Autodesk Fusion 360 part; units mm, degrees
(part 3 of 15)
  spline S34 degree 5 poles (-13.0691, -22.8361) (-13.0745, -22.8455) (-13.085, -22.8643) (-13.1, -22.893) (-13.1188, -22.9319) (-13.1404, -22.9814) (-13.1608, -23.0315) (-13.1803, -23.0821) (-13.1994, -23.133) (-13.2182, -23.1839) (-13.2367, -23.2351) (-13.2548, -23.2864) (-13.2724, -23.338) (-13.2894, -23.3899) (-13.3057, -23.4421) (-13.3214, -23.4946) (-13.3366, -23.5473) (-13.3514, -23.6002) (-13.3658, -23.6533) (-13.3798, -23.7066) (-13.3935, -23.76) (-13.4069, -23.8135) (-13.4198, -23.8673) (-13.4324, -23.9212) (-13.4445, -23.9753) (-13.4563, -24.0295) (-13.4677, -24.0839) (-13.4788, -24.1385) (-13.4895, -24.1932) (-13.4999, -24.248) (-13.51, -24.3029) (-13.5197, -24.358) (-13.5291, -24.4132) (-13.5382, -24.4686) (-13.547, -24.524) (-13.5555, -24.5796) (-13.5636, -24.6353) (-13.5714, -24.6912) (-13.579, -24.7471) (-13.5862, -24.8032) (-13.5932, -24.8593) (-13.5998, -24.9156) (-13.6062, -24.972) (-13.6123, -25.0284) (-13.618, -25.085) (-13.6235, -25.1417) (-13.6288, -25.1985) (-13.6337, -25.2553) (-13.6383, -25.3123) (-13.6427, -25.3694) (-13.6468, -25.4265) (-13.6507, -25.4838) (-13.6542, -25.5411) (-13.6575, -25.5985) (-13.6606, -25.656) (-13.6633, -25.7136) (-13.6659, -25.7712) (-13.6681, -25.829) (-13.6701, -25.8868) (-13.6718, -25.9447) (-13.6733, -26.0027) (-13.6745, -26.0607) (-13.6754, -26.1188) (-13.6761, -26.177) (-13.6766, -26.2353) (-13.6768, -26.2936) (-13.6767, -26.3521) (-13.6765, -26.4105) (-13.6759, -26.4691) (-13.6751, -26.5277) (-13.6741, -26.5863) (-13.6731, -26.6333) (-13.6722, -26.6686) (-13.6715, -26.6921) (-13.6712, -26.7039) knots 0 0 0 0 0 0 0.01428571 0.02857143 0.04285714 0.05714286 0.07142857 0.08571429 0.1 0.11428571 0.12857143 0.14285714 0.15714286 0.17142857 0.18571429 0.2 0.21428571 0.22857143 0.24285714 0.25714286 0.27142857 0.28571429 0.3 0.31428571 0.32857143 0.34285714 0.35714286 0.37142857 0.38571429 0.4 0.41428571 0.42857143 0.44285714 0.45714286 0.47142857 0.48571429 0.5 0.51428571 0.52857143 0.54285714 0.55714286 0.57142857 0.58571429 0.6 0.61428571 0.62857143 0.64285714 0.65714286 0.67142857 0.68571429 0.7 0.71428571 0.72857143 0.74285714 0.75714286 0.77142857 0.78571429 0.8 0.81428571 0.82857143 0.84285714 0.85714286 0.87142857 0.88571429 0.9 0.91428571 0.92857143 0.94285714 0.95714286 0.97142857 0.98571429 1 1 1 1 1 1
  arc A36 (-13.6712, -26.7039) -> (-12.3541, -27.3382) centre (0, 0) ccw
  spline S35 degree 5 poles (-9.7055, -24.4559) (-9.7095, -24.466) (-9.7177, -24.4859) (-9.7307, -24.5156) (-9.7494, -24.5545) (-9.7746, -24.6023) (-9.8012, -24.6494) (-9.8286, -24.6963) (-9.8564, -24.7429) (-9.8845, -24.7894) (-9.9129, -24.8357) (-9.9418, -24.8819) (-9.9712, -24.9278) (-10.0012, -24.9734) (-10.0318, -25.0187) (-10.0631, -25.0637) (-10.0948, -25.1085) (-10.127, -25.153) (-10.1595, -25.1974) (-10.1924, -25.2416) (-10.2256, -25.2856) (-10.2591, -25.3294) (-10.2931, -25.3731) (-10.3274, -25.4165) (-10.3621, -25.4597) (-10.3972, -25.5027) (-10.4326, -25.5456) (-10.4683, -25.5882) (-10.5044, -25.6307) (-10.5408, -25.673) (-10.5775, -25.7151) (-10.6145, -25.7571) (-10.6518, -25.7989) (-10.6894, -25.8405) (-10.7273, -25.882) (-10.7654, -25.9232) (-10.8039, -25.9643) (-10.8427, -26.0053) (-10.8817, -26.0461) (-10.921, -26.0867) (-10.9606, -26.1271) (-11.0004, -26.1674) (-11.0406, -26.2075) (-11.0809, -26.2475) (-11.1216, -26.2873) (-11.1624, -26.3269) (-11.2036, -26.3664) (-11.245, -26.4057) (-11.2866, -26.4449) (-11.3285, -26.4839) (-11.3706, -26.5227) (-11.4129, -26.5614) (-11.4555, -26.5999) (-11.4984, -26.6383) (-11.5414, -26.6765) (-11.5847, -26.7146) (-11.6282, -26.7525) (-11.672, -26.7902) (-11.716, -26.8279) (-11.7601, -26.8653) (-11.8046, -26.9026) (-11.8492, -26.9397) (-11.894, -26.9767) (-11.9391, -27.0136) (-11.9844, -27.0502) (-12.0299, -27.0868) (-12.0755, -27.1231) (-12.1215, -27.1594) (-12.1676, -27.1954) (-12.2139, -27.2314) (-12.2604, -27.2671) (-12.2978, -27.2956) (-12.3259, -27.3169) (-12.3447, -27.3311) (-12.3541, -27.3382) knots 0 0 0 0 0 0 0.01428571 0.02857143 0.04285714 0.05714286 0.07142857 0.08571429 0.1 0.11428571 0.12857143 0.14285714 0.15714286 0.17142857 0.18571429 0.2 0.21428571 0.22857143 0.24285714 0.25714286 0.27142857 0.28571429 0.3 0.31428571 0.32857143 0.34285714 0.35714286 0.37142857 0.38571429 0.4 0.41428571 0.42857143 0.44285714 0.45714286 0.47142857 0.48571429 0.5 0.51428571 0.52857143 0.54285714 0.55714286 0.57142857 0.58571429 0.6 0.61428571 0.62857143 0.64285714 0.65714286 0.67142857 0.68571429 0.7 0.71428571 0.72857143 0.74285714 0.75714286 0.77142857 0.78571429 0.8 0.81428571 0.82857143 0.84285714 0.85714286 0.87142857 0.88571429 0.9 0.91428571 0.92857143 0.94285714 0.95714286 0.97142857 0.98571429 1 1 1 1 1 1
  line L35 (-9.7055, -24.4559) -> (-9.4748, -23.8746)
  arc A37 (-9.4748, -23.8746) -> (-7.4779, -24.5734) centre (0, 0) ccw
  line L36 (-7.4779, -24.5734) -> (-7.6599, -25.1717)
  spline S36 degree 5 poles (-7.6599, -25.1717) (-7.6631, -25.182) (-7.6691, -25.2028) (-7.6774, -25.2341) (-7.6871, -25.2761) (-7.6971, -25.3292) (-7.7058, -25.3826) (-7.7136, -25.4363) (-7.7209, -25.4901) (-7.7279, -25.544) (-7.7346, -25.598) (-7.7408, -25.6521) (-7.7465, -25.7063) (-7.7514, -25.7606) (-7.7557, -25.8152) (-7.7594, -25.8698) (-7.7625, -25.9246) (-7.7651, -25.9795) (-7.7673, -26.0345) (-7.7692, -26.0895) (-7.7706, -26.1446) (-7.7717, -26.1998) (-7.7724, -26.2551) (-7.7726, -26.3104) (-7.7725, -26.3659) (-7.7719, -26.4214) (-7.7709, -26.4769) (-7.7695, -26.5326) (-7.7678, -26.5883) (-7.7657, -26.644) (-7.7633, -26.6999) (-7.7606, -26.7557) (-7.7575, -26.8117) (-7.754, -26.8676) (-7.7502, -26.9237) (-7.7461, -26.9797) (-7.7417, -27.0359) (-7.7369, -27.092) (-7.7318, -27.1483) (-7.7264, -27.2045) (-7.7206, -27.2608) (-7.7146, -27.3172) (-7.7083, -27.3735) (-7.7016, -27.4299) (-7.6947, -27.4864) (-7.6874, -27.5429) (-7.6799, -27.5994) (-7.672, -27.6559) (-7.6639, -27.7125) (-7.6555, -27.7691) (-7.6468, -27.8257) (-7.6378, -27.8824) (-7.6285, -27.9391) (-7.6189, -27.9958) (-7.6091, -28.0525) (-7.599, -28.1093) (-7.5886, -28.166) (-7.5779, -28.2228) (-7.567, -28.2796) (-7.5558, -28.3365) (-7.5443, -28.3933) (-7.5326, -28.4502) (-7.5206, -28.5071) (-7.5083, -28.564) (-7.4958, -28.6209) (-7.483, -28.6778) (-7.47, -28.7347) (-7.4567, -28.7917) (-7.4431, -28.8486) (-7.4293, -28.9056) (-7.4152, -28.9625) (-7.4038, -29.0081) (-7.3951, -29.0423) (-7.3892, -29.0651) (-7.3863, -29.0765) knots 0 0 0 0 0 0 0.01428571 0.02857143 0.04285714 0.05714286 0.07142857 0.08571429 0.1 0.11428571 0.12857143 0.14285714 0.15714286 0.17142857 0.18571429 0.2 0.21428571 0.22857143 0.24285714 0.25714286 0.27142857 0.28571429 0.3 0.31428571 0.32857143 0.34285714 0.35714286 0.37142857 0.38571429 0.4 0.41428571 0.42857143 0.44285714 0.45714286 0.47142857 0.48571429 0.5 0.51428571 0.52857143 0.54285714 0.55714286 0.57142857 0.58571429 0.6 0.61428571 0.62857143 0.64285714 0.65714286 0.67142857 0.68571429 0.7 0.71428571 0.72857143 0.74285714 0.75714286 0.77142857 0.78571429 0.8 0.81428571 0.82857143 0.84285714 0.85714286 0.87142857 0.88571429 0.9 0.91428571 0.92857143 0.94285714 0.95714286 0.97142857 0.98571429 1 1 1 1 1 1
  arc A38 (-7.3863, -29.0765) -> (-5.961, -29.4018) centre (0, 0) ccw
  spline S37 degree 5 poles (-4.0202, -26.0024) (-4.0219, -26.0131) (-4.0254, -26.0344) (-4.0315, -26.0662) (-4.0411, -26.1083) (-4.055, -26.1605) (-4.0704, -26.2124) (-4.0867, -26.2641) (-4.1034, -26.3158) (-4.1205, -26.3674) (-4.1379, -26.4189) (-4.1558, -26.4703) (-4.1742, -26.5216) (-4.1933, -26.5728) (-4.2131, -26.6237) (-4.2336, -26.6746) (-4.2545, -26.7253) (-4.276, -26.7759) (-4.2978, -26.8263) (-4.32, -26.8767) (-4.3426, -26.927) (-4.3656, -26.9772) (-4.389, -27.0273) (-4.4128, -27.0773) (-4.437, -27.1272) (-4.4616, -27.1769) (-4.4866, -27.2266) (-4.512, -27.2761) (-4.5377, -27.3255) (-4.5637, -27.3749) (-4.5901, -27.4241) (-4.6168, -27.4733) (-4.6439, -27.5223) (-4.6713, -27.5712) (-4.699, -27.6201) (-4.7271, -27.6688) (-4.7554, -27.7175) (-4.7841, -27.766) (-4.8131, -27.8144) (-4.8424, -27.8628) (-4.872, -27.911) (-4.9018, -27.9591) (-4.932, -28.0072) (-4.9625, -28.0551) (-4.9932, -28.103) (-5.0243, -28.1507) (-5.0556, -28.1983) (-5.0872, -28.2459) (-5.1191, -28.2933) (-5.1512, -28.3407) (-5.1836, -28.3879) (-5.2163, -28.4351) (-5.2493, -28.4821) (-5.2825, -28.529) (-5.316, -28.5759) (-5.3497, -28.6226) (-5.3837, -28.6693) (-5.418, -28.7158) (-5.4525, -28.7623) (-5.4872, -28.8086) (-5.5222, -28.8548) (-5.5574, -28.901) (-5.5929, -28.947) (-5.6287, -28.993) (-5.6647, -29.0388) (-5.7009, -29.0845) (-5.7373, -29.1302) (-5.774, -29.1757) (-5.8109, -29.2211) (-5.8481, -29.2665) (-5.8855, -29.3117) (-5.9156, -29.3478) (-5.9383, -29.3748) (-5.9534, -29.3928) (-5.961, -29.4018) knots 0 0 0 0 0 0 0.01428571 0.02857143 0.04285714 0.05714286 0.07142857 0.08571429 0.1 0.11428571 0.12857143 0.14285714 0.15714286 0.17142857 0.18571429 0.2 0.21428571 0.22857143 0.24285714 0.25714286 0.27142857 0.28571429 0.3 0.31428571 0.32857143 0.34285714 0.35714286 0.37142857 0.38571429 0.4 0.41428571 0.42857143 0.44285714 0.45714286 0.47142857 0.48571429 0.5 0.51428571 0.52857143 0.54285714 0.55714286 0.57142857 0.58571429 0.6 0.61428571 0.62857143 0.64285714 0.65714286 0.67142857 0.68571429 0.7 0.71428571 0.72857143 0.74285714 0.75714286 0.77142857 0.78571429 0.8 0.81428571 0.82857143 0.84285714 0.85714286 0.87142857 0.88571429 0.9 0.91428571 0.92857143 0.94285714 0.95714286 0.97142857 0.98571429 1 1 1 1 1 1
  line L37 (-4.0202, -26.0024) -> (-3.9247, -25.3844)
  arc A39 (-3.9247, -25.3844) -> (-1.8223, -25.6213) centre (0, 0) ccw
  line L38 (-1.8223, -25.6213) -> (-1.8667, -26.2451)
  spline S38 degree 5 poles (-1.8667, -26.2451) (-1.8674, -26.2559) (-1.8687, -26.2774) (-1.8698, -26.3098) (-1.8699, -26.3529) (-1.8679, -26.4069) (-1.8644, -26.461) (-1.8601, -26.515) (-1.8552, -26.5691) (-1.8501, -26.6232) (-1.8446, -26.6773) (-1.8386, -26.7314) (-1.8321, -26.7855) (-1.8248, -26.8396) (-1.8169, -26.8937) (-1.8082, -26.9478) (-1.7991, -27.0019) (-1.7894, -27.056) (-1.7794, -27.1101) (-1.7689, -27.1642) (-1.7581, -27.2182) (-1.7469, -27.2723) (-1.7352, -27.3263) (-1.7231, -27.3803) (-1.7106, -27.4343) (-1.6977, -27.4883) (-1.6844, -27.5423) (-1.6707, -27.5962) (-1.6566, -27.6502) (-1.6422, -27.7041) (-1.6274, -27.7579) (-1.6123, -27.8118) (-1.5968, -27.8656) (-1.581, -27.9194) (-1.5648, -27.9732) (-1.5483, -28.027) (-1.5315, -28.0807) (-1.5143, -28.1344) (-1.4969, -28.1881) (-1.4791, -28.2417) (-1.461, -28.2953) (-1.4425, -28.3489) (-1.4238, -28.4025) (-1.4048, -28.456) (-1.3854, -28.5095) (-1.3658, -28.5629) (-1.3459, -28.6163) (-1.3256, -28.6697) (-1.3051, -28.7231) (-1.2843, -28.7764) (-1.2632, -28.8296) (-1.2418, -28.8829) (-1.2202, -28.9361) (-1.1983, -28.9892) (-1.176, -29.0423) (-1.1536, -29.0954) (-1.1308, -29.1485) (-1.1078, -29.2015) (-1.0845, -29.2544) (-1.0609, -29.3073) (-1.0371, -29.3602) (-1.013, -29.413) (-0.9886, -29.4658) (-0.964, -29.5186) (-0.9391, -29.5712) (-0.914, -29.6239) (-0.8886, -29.6765) (-0.863, -29.729) (-0.8371, -29.7816) (-0.8109, -29.834) (-0.7845, -29.8864) (-0.7632, -29.9283) (-0.7471, -29.9597) (-0.7364, -29.9806) (-0.731, -29.9911) knots 0 0 0 0 0 0 0.01428571 0.02857143 0.04285714 0.05714286 0.07142857 0.08571429 0.1 0.11428571 0.12857143 0.14285714 0.15714286 0.17142857 0.18571429 0.2 0.21428571 0.22857143 0.24285714 0.25714286 0.27142857 0.28571429 0.3 0.31428571 0.32857143 0.34285714 0.35714286 0.37142857 0.38571429 0.4 0.41428571 0.42857143 0.44285714 0.45714286 0.47142857 0.48571429 0.5 0.51428571 0.52857143 0.54285714 0.55714286 0.57142857 0.58571429 0.6 0.61428571 0.62857143 0.64285714 0.65714286 0.67142857 0.68571429 0.7 0.71428571 0.72857143 0.74285714 0.75714286 0.77142857 0.78571429 0.8 0.81428571 0.82857143 0.84285714 0.85714286 0.87142857 0.88571429 0.9 0.91428571 0.92857143 0.94285714 0.95714286 0.97142857 0.98571429 1 1 1 1 1 1
  arc A40 (-0.731, -29.9911) -> (0.731, -29.9911) centre (0, 0) ccw
  spline S39 degree 5 poles (1.8667, -26.2451) (1.8674, -26.2559) (1.8687, -26.2774) (1.8698, -26.3098) (1.8699, -26.3529) (1.8679, -26.4069) (1.8644, -26.461) (1.8601, -26.515) (1.8552, -26.5691) (1.8501, -26.6232) (1.8446, -26.6773) (1.8386, -26.7314) (1.8321, -26.7855) (1.8248, -26.8396) (1.8169, -26.8937) (1.8082, -26.9478) (1.7991, -27.0019) (1.7894, -27.056) (1.7794, -27.1101) (1.7689, -27.1642) (1.7581, -27.2182) (1.7469, -27.2723) (1.7352, -27.3263) (1.7231, -27.3803) (1.7106, -27.4343) (1.6977, -27.4883) (1.6844, -27.5423) (1.6707, -27.5962) (1.6566, -27.6502) (1.6422, -27.7041) (1.6274, -27.7579) (1.6123, -27.8118) (1.5968, -27.8656) (1.581, -27.9194) (1.5648, -27.9732) (1.5483, -28.027) (1.5315, -28.0807) (1.5143, -28.1344) (1.4969, -28.1881) (1.4791, -28.2417) (1.461, -28.2953) (1.4425, -28.3489) (1.4238, -28.4025) (1.4048, -28.456) (1.3854, -28.5095) (1.3658, -28.5629) (1.3459, -28.6163) (1.3256, -28.6697) (1.3051, -28.7231) (1.2843, -28.7764) (1.2632, -28.8296) (1.2418, -28.8829) (1.2202, -28.9361) (1.1983, -28.9892) (1.176, -29.0423) (1.1536, -29.0954) (1.1308, -29.1485) (1.1078, -29.2015) (1.0845, -29.2544) (1.0609, -29.3073) (1.0371, -29.3602) (1.013, -29.413) (0.9886, -29.4658) (0.964, -29.5186) (0.9391, -29.5712) (0.914, -29.6239) (0.8886, -29.6765) (0.863, -29.729) (0.8371, -29.7816) (0.8109, -29.834) (0.7845, -29.8864) (0.7632, -29.9283) (0.7471, -29.9597) (0.7364, -29.9806) (0.731, -29.9911) knots 0 0 0 0 0 0 0.01428571 0.02857143 0.04285714 0.05714286 0.07142857 0.08571429 0.1 0.11428571 0.12857143 0.14285714 0.15714286 0.17142857 0.18571429 0.2 0.21428571 0.22857143 0.24285714 0.25714286 0.27142857 0.28571429 0.3 0.31428571 0.32857143 0.34285714 0.35714286 0.37142857 0.38571429 0.4 0.41428571 0.42857143 0.44285714 0.45714286 0.47142857 0.48571429 0.5 0.51428571 0.52857143 0.54285714 0.55714286 0.57142857 0.58571429 0.6 0.61428571 0.62857143 0.64285714 0.65714286 0.67142857 0.68571429 0.7 0.71428571 0.72857143 0.74285714 0.75714286 0.77142857 0.78571429 0.8 0.81428571 0.82857143 0.84285714 0.85714286 0.87142857 0.88571429 0.9 0.91428571 0.92857143 0.94285714 0.95714286 0.97142857 0.98571429 1 1 1 1 1 1
  line L39 (1.8667, -26.2451) -> (1.8223, -25.6213)
  arc A41 (1.8223, -25.6213) -> (3.9247, -25.3844) centre (0, 0) ccw
  line L40 (3.9247, -25.3844) -> (4.0202, -26.0024)
  spline S40 degree 5 poles (4.0202, -26.0024) (4.0219, -26.0131) (4.0254, -26.0344) (4.0315, -26.0662) (4.0411, -26.1083) (4.055, -26.1605) (4.0704, -26.2124) (4.0867, -26.2641) (4.1034, -26.3158) (4.1205, -26.3674) (4.1379, -26.4189) (4.1558, -26.4703) (4.1742, -26.5216) (4.1933, -26.5728) (4.2131, -26.6237) (4.2336, -26.6746) (4.2545, -26.7253) (4.276, -26.7759) (4.2978, -26.8263) (4.32, -26.8767) (4.3426, -26.927) (4.3656, -26.9772) (4.389, -27.0273) (4.4128, -27.0773) (4.437, -27.1272) (4.4616, -27.1769) (4.4866, -27.2266) (4.512, -27.2761) (4.5377, -27.3255) (4.5637, -27.3749) (4.5901, -27.4241) (4.6168, -27.4733) (4.6439, -27.5223) (4.6713, -27.5712) (4.699, -27.6201) (4.7271, -27.6688) (4.7554, -27.7175) (4.7841, -27.766) (4.8131, -27.8144) (4.8424, -27.8628) (4.872, -27.911) (4.9018, -27.9591) (4.932, -28.0072) (4.9625, -28.0551) (4.9932, -28.103) (5.0243, -28.1507) (5.0556, -28.1983) (5.0872, -28.2459) (5.1191, -28.2933) (5.1512, -28.3407) (5.1836, -28.3879) (5.2163, -28.4351) (5.2493, -28.4821) (5.2825, -28.529) (5.316, -28.5759) (5.3497, -28.6226) (5.3837, -28.6693) (5.418, -28.7158) (5.4525, -28.7623) (5.4872, -28.8086) (5.5222, -28.8548) (5.5574, -28.901) (5.5929, -28.947) (5.6287, -28.993) (5.6647, -29.0388) (5.7009, -29.0845) (5.7373, -29.1302) (5.774, -29.1757) (5.8109, -29.2211) (5.8481, -29.2665) (5.8855, -29.3117) (5.9156, -29.3478) (5.9383, -29.3748) (5.9534, -29.3928) (5.961, -29.4018) knots 0 0 0 0 0 0 0.01428571 0.02857143 0.04285714 0.05714286 0.07142857 0.08571429 0.1 0.11428571 0.12857143 0.14285714 0.15714286 0.17142857 0.18571429 0.2 0.21428571 0.22857143 0.24285714 0.25714286 0.27142857 0.28571429 0.3 0.31428571 0.32857143 0.34285714 0.35714286 0.37142857 0.38571429 0.4 0.41428571 0.42857143 0.44285714 0.45714286 0.47142857 0.48571429 0.5 0.51428571 0.52857143 0.54285714 0.55714286 0.57142857 0.58571429 0.6 0.61428571 0.62857143 0.64285714 0.65714286 0.67142857 0.68571429 0.7 0.71428571 0.72857143 0.74285714 0.75714286 0.77142857 0.78571429 0.8 0.81428571 0.82857143 0.84285714 0.85714286 0.87142857 0.88571429 0.9 0.91428571 0.92857143 0.94285714 0.95714286 0.97142857 0.98571429 1 1 1 1 1 1
  arc A42 (5.961, -29.4018) -> (7.3863, -29.0765) centre (0, 0) ccw
  spline S41 degree 5 poles (7.6599, -25.1717) (7.6631, -25.182) (7.6691, -25.2028) (7.6774, -25.2341) (7.6871, -25.2761) (7.6971, -25.3292) (7.7058, -25.3826) (7.7136, -25.4363) (7.7209, -25.4901) (7.7279, -25.544) (7.7346, -25.598) (7.7408, -25.6521) (7.7465, -25.7063) (7.7514, -25.7606) (7.7557, -25.8152) (7.7594, -25.8698) (7.7625, -25.9246) (7.7651, -25.9795) (7.7673, -26.0345) (7.7692, -26.0895) (7.7706, -26.1446) (7.7717, -26.1998) (7.7724, -26.2551) (7.7726, -26.3104) (7.7725, -26.3659) (7.7719, -26.4214) (7.7709, -26.4769) (7.7695, -26.5326) (7.7678, -26.5883) (7.7657, -26.644) (7.7633, -26.6999) (7.7606, -26.7557) (7.7575, -26.8117) (7.754, -26.8676) (7.7502, -26.9237) (7.7461, -26.9797) (7.7417, -27.0359) (7.7369, -27.092) (7.7318, -27.1483) (7.7264, -27.2045) (7.7206, -27.2608) (7.7146, -27.3172) (7.7083, -27.3735) (7.7016, -27.4299) (7.6947, -27.4864) (7.6874, -27.5429) (7.6799, -27.5994) (7.672, -27.6559) (7.6639, -27.7125) (7.6555, -27.7691) (7.6468, -27.8257) (7.6378, -27.8824) (7.6285, -27.9391) (7.6189, -27.9958) (7.6091, -28.0525) (7.599, -28.1093) (7.5886, -28.166) (7.5779, -28.2228) (7.567, -28.2796) (7.5558, -28.3365) (7.5443, -28.3933) (7.5326, -28.4502) (7.5206, -28.5071) (7.5083, -28.564) (7.4958, -28.6209) (7.483, -28.6778) (7.47, -28.7347) (7.4567, -28.7917) (7.4431, -28.8486) (7.4293, -28.9056) (7.4152, -28.9625) (7.4038, -29.0081) (7.3951, -29.0423) (7.3892, -29.0651) (7.3863, -29.0765) knots 0 0 0 0 0 0 0.01428571 0.02857143 0.04285714 0.05714286 0.07142857 0.08571429 0.1 0.11428571 0.12857143 0.14285714 0.15714286 0.17142857 0.18571429 0.2 0.21428571 0.22857143 0.24285714 0.25714286 0.27142857 0.28571429 0.3 0.31428571 0.32857143 0.34285714 0.35714286 0.37142857 0.38571429 0.4 0.41428571 0.42857143 0.44285714 0.45714286 0.47142857 0.48571429 0.5 0.51428571 0.52857143 0.54285714 0.55714286 0.57142857 0.58571429 0.6 0.61428571 0.62857143 0.64285714 0.65714286 0.67142857 0.68571429 0.7 0.71428571 0.72857143 0.74285714 0.75714286 0.77142857 0.78571429 0.8 0.81428571 0.82857143 0.84285714 0.85714286 0.87142857 0.88571429 0.9 0.91428571 0.92857143 0.94285714 0.95714286 0.97142857 0.98571429 1 1 1 1 1 1
  line L41 (7.6599, -25.1717) -> (7.4779, -24.5734)
  arc A43 (7.4779, -24.5734) -> (9.4748, -23.8746) centre (0, 0) ccw
  line L42 (9.4748, -23.8746) -> (9.7055, -24.4559)
  spline S42 degree 5 poles (9.7055, -24.4559) (9.7095, -24.466) (9.7177, -24.4859) (9.7307, -24.5156) (9.7494, -24.5545) (9.7746, -24.6023) (9.8012, -24.6494) (9.8286, -24.6963) (9.8564, -24.7429) (9.8845, -24.7894) (9.9129, -24.8357) (9.9418, -24.8819) (9.9712, -24.9278) (10.0012, -24.9734) (10.0318, -25.0187) (10.0631, -25.0637) (10.0948, -25.1085) (10.127, -25.153) (10.1595, -25.1974) (10.1924, -25.2416) (10.2256, -25.2856) (10.2591, -25.3294) (10.2931, -25.3731) (10.3274, -25.4165) (10.3621, -25.4597) (10.3972, -25.5027) (10.4326, -25.5456) (10.4683, -25.5882) (10.5044, -25.6307) (10.5408, -25.673) (10.5775, -25.7151) (10.6145, -25.7571) (10.6518, -25.7989) (10.6894, -25.8405) (10.7273, -25.882) (10.7654, -25.9232) (10.8039, -25.9643) (10.8427, -26.0053) (10.8817, -26.0461) (10.921, -26.0867) (10.9606, -26.1271) (11.0004, -26.1674) (11.0406, -26.2075) (11.0809, -26.2475) (11.1216, -26.2873) (11.1624, -26.3269) (11.2036, -26.3664) (11.245, -26.4057) (11.2866, -26.4449) (11.3285, -26.4839) (11.3706, -26.5227) (11.4129, -26.5614) (11.4555, -26.5999) (11.4984, -26.6383) (11.5414, -26.6765) (11.5847, -26.7146) (11.6282, -26.7525) (11.672, -26.7902) (11.716, -26.8279) (11.7601, -26.8653) (11.8046, -26.9026) (11.8492, -26.9397) (11.894, -26.9767) (11.9391, -27.0136) (11.9844, -27.0502) (12.0299, -27.0868) (12.0755, -27.1231) (12.1215, -27.1594) (12.1676, -27.1954) (12.2139, -27.2314) (12.2604, -27.2671) (12.2978, -27.2956) (12.3259, -27.3169) (12.3447, -27.3311) (12.3541, -27.3382) knots 0 0 0 0 0 0 0.01428571 0.02857143 0.04285714 0.05714286 0.07142857 0.08571429 0.1 0.11428571 0.12857143 0.14285714 0.15714286 0.17142857 0.18571429 0.2 0.21428571 0.22857143 0.24285714 0.25714286 0.27142857 0.28571429 0.3 0.31428571 0.32857143 0.34285714 0.35714286 0.37142857 0.38571429 0.4 0.41428571 0.42857143 0.44285714 0.45714286 0.47142857 0.48571429 0.5 0.51428571 0.52857143 0.54285714 0.55714286 0.57142857 0.58571429 0.6 0.61428571 0.62857143 0.64285714 0.65714286 0.67142857 0.68571429 0.7 0.71428571 0.72857143 0.74285714 0.75714286 0.77142857 0.78571429 0.8 0.81428571 0.82857143 0.84285714 0.85714286 0.87142857 0.88571429 0.9 0.91428571 0.92857143 0.94285714 0.95714286 0.97142857 0.98571429 1 1 1 1 1 1
  arc A44 (12.3541, -27.3382) -> (13.6712, -26.7039) centre (0, 0) ccw
  spline S43 degree 5 poles (13.0691, -22.8361) (13.0745, -22.8455) (13.085, -22.8643) (13.1, -22.893) (13.1188, -22.9319) (13.1404, -22.9814) (13.1608, -23.0315) (13.1803, -23.0821) (13.1994, -23.133) (13.2182, -23.1839) (13.2367, -23.2351) (13.2548, -23.2864) (13.2724, -23.338) (13.2894, -23.3899) (13.3057, -23.4421) (13.3214, -23.4946) (13.3366, -23.5473) (13.3514, -23.6002) (13.3658, -23.6533) (13.3798, -23.7066) (13.3935, -23.76) (13.4069, -23.8135) (13.4198, -23.8673) (13.4324, -23.9212) (13.4445, -23.9753) (13.4563, -24.0295) (13.4677, -24.0839) (13.4788, -24.1385) (13.4895, -24.1932) (13.4999, -24.248) (13.51, -24.3029) (13.5197, -24.358) (13.5291, -24.4132) (13.5382, -24.4686) (13.547, -24.524) (13.5555, -24.5796) (13.5636, -24.6353) (13.5714, -24.6912) (13.579, -24.7471) (13.5862, -24.8032) (13.5932, -24.8593) (13.5998, -24.9156) (13.6062, -24.972) (13.6123, -25.0284) (13.618, -25.085) (13.6235, -25.1417) (13.6288, -25.1985) (13.6337, -25.2553) (13.6383, -25.3123) (13.6427, -25.3694) (13.6468, -25.4265) (13.6507, -25.4838) (13.6542, -25.5411) (13.6575, -25.5985) (13.6606, -25.656) (13.6633, -25.7136) (13.6659, -25.7712) (13.6681, -25.829) (13.6701, -25.8868) (13.6718, -25.9447) (13.6733, -26.0027) (13.6745, -26.0607) (13.6754, -26.1188) (13.6761, -26.177) (13.6766, -26.2353) (13.6768, -26.2936) (13.6767, -26.3521) (13.6765, -26.4105) (13.6759, -26.4691) (13.6751, -26.5277) (13.6741, -26.5863) (13.6731, -26.6333) (13.6722, -26.6686) (13.6715, -26.6921) (13.6712, -26.7039) knots 0 0 0 0 0 0 0.01428571 0.02857143 0.04285714 0.05714286 0.07142857 0.08571429 0.1 0.11428571 0.12857143 0.14285714 0.15714286 0.17142857 0.18571429 0.2 0.21428571 0.22857143 0.24285714 0.25714286 0.27142857 0.28571429 0.3 0.31428571 0.32857143 0.34285714 0.35714286 0.37142857 0.38571429 0.4 0.41428571 0.42857143 0.44285714 0.45714286 0.47142857 0.48571429 0.5 0.51428571 0.52857143 0.54285714 0.55714286 0.57142857 0.58571429 0.6 0.61428571 0.62857143 0.64285714 0.65714286 0.67142857 0.68571429 0.7 0.71428571 0.72857143 0.74285714 0.75714286 0.77142857 0.78571429 0.8 0.81428571 0.82857143 0.84285714 0.85714286 0.87142857 0.88571429 0.9 0.91428571 0.92857143 0.94285714 0.95714286 0.97142857 0.98571429 1 1 1 1 1 1
  line L43 (13.0691, -22.8361) -> (12.7585, -22.2933)
  arc A45 (12.7585, -22.2933) -> (14.5499, -21.1677) centre (0, 0) ccw
  line L44 (14.5499, -21.1677) -> (14.9041, -21.6831)
  spline S44 degree 5 poles (14.9041, -21.6831) (14.9103, -21.692) (14.9227, -21.7096) (14.942, -21.7356) (14.9689, -21.7694) (15.0041, -21.8104) (15.0405, -21.8505) (15.0776, -21.89) (15.1151, -21.9293) (15.1528, -21.9683) (15.1909, -22.0072) (15.2293, -22.0458) (15.2681, -22.084) (15.3075, -22.1218) (15.3475, -22.1592) (15.388, -22.1961) (15.4289, -22.2327) (15.4701, -22.2689) (15.5117, -22.3049) (15.5536, -22.3407) (15.5958, -22.3762) (15.6382, -22.4115) (15.681, -22.4465) (15.7242, -22.4812) (15.7676, -22.5156) (15.8114, -22.5497) (15.8554, -22.5836) (15.8998, -22.6172) (15.9444, -22.6506) (15.9893, -22.6838) (16.0344, -22.7167) (16.0798, -22.7494) (16.1255, -22.7818) (16.1714, -22.814) (16.2176, -22.846) (16.264, -22.8777) (16.3107, -22.9093) (16.3576, -22.9405) (16.4047, -22.9716) (16.452, -23.0025) (16.4996, -23.0331) (16.5474, -23.0635) (16.5955, -23.0937) (16.6437, -23.1237) (16.6922, -23.1534) (16.7409, -23.183) (16.7897, -23.2123) (16.8388, -23.2414) (16.8881, -23.2703) (16.9377, -23.299) (16.9874, -23.3275) (17.0373, -23.3558) (17.0874, -23.3839) (17.1377, -23.4118) (17.1881, -23.4395) (17.2388, -23.467) (17.2897, -23.4942) (17.3407, -23.5213) (17.392, -23.5482) (17.4434, -23.5749) (17.495, -23.6013) (17.5468, -23.6276) (17.5987, -23.6537) (17.6508, -23.6796) (17.7031, -23.7053) (17.7556, -23.7308) (17.8083, -23.7561) (17.8611, -23.7812) (17.914, -23.8061) (17.9672, -23.8308) (18.0205, -23.8553) (18.0633, -23.8748) (18.0954, -23.8893) (18.1169, -23.8989) (18.1277, -23.9037) knots 0 0 0 0 0 0 0.01428571 0.02857143 0.04285714 0.05714286 0.07142857 0.08571429 0.1 0.11428571 0.12857143 0.14285714 0.15714286 0.17142857 0.18571429 0.2 0.21428571 0.22857143 0.24285714 0.25714286 0.27142857 0.28571429 0.3 0.31428571 0.32857143 0.34285714 0.35714286 0.37142857 0.38571429 0.4 0.41428571 0.42857143 0.44285714 0.45714286 0.47142857 0.48571429 0.5 0.51428571 0.52857143 0.54285714 0.55714286 0.57142857 0.58571429 0.6 0.61428571 0.62857143 0.64285714 0.65714286 0.67142857 0.68571429 0.7 0.71428571 0.72857143 0.74285714 0.75714286 0.77142857 0.78571429 0.8 0.81428571 0.82857143 0.84285714 0.85714286 0.87142857 0.88571429 0.9 0.91428571 0.92857143 0.94285714 0.95714286 0.97142857 0.98571429 1 1 1 1 1 1
  arc A46 (18.1277, -23.9037) -> (19.2706, -22.9922) centre (0, 0) ccw
  spline S45 degree 5 poles (17.823, -19.3554) (17.8303, -19.3633) (17.8447, -19.3794) (17.8658, -19.404) (17.8927, -19.4377) (17.9248, -19.4812) (17.9558, -19.5255) (17.9861, -19.5705) (18.016, -19.6158) (18.0457, -19.6613) (18.0752, -19.7071) (18.1042, -19.7531) (18.1329, -19.7995) (18.1609, -19.8463) (18.1884, -19.8936) (18.2154, -19.9412) (18.242, -19.9893) (18.2682, -20.0376) (18.294, -20.0861) (18.3196, -20.1349) (18.3448, -20.1839) (18.3698, -20.2332) (18.3943, -20.2827) (18.4186, -20.3324) (18.4425, -20.3825) (18.466, -20.4327) (18.4892, -20.4832) (18.5121, -20.534) (18.5348, -20.5849) (18.5571, -20.636) (18.5792, -20.6874) (18.6009, -20.7389) (18.6224, -20.7906) (18.6436, -20.8426) (18.6645, -20.8947) (18.6851, -20.947) (18.7054, -20.9995) (18.7255, -21.0522) (18.7453, -21.105) (18.7648, -21.1581) (18.7841, -21.2113) (18.8031, -21.2647) (18.8218, -21.3182) (18.8403, -21.3719) (18.8585, -21.4258) (18.8765, -21.4798) (18.8942, -21.534) (18.9117, -21.5884) (18.9289, -21.6429) (18.9459, -21.6975) (18.9626, -21.7523) (18.9791, -21.8073) (18.9953, -21.8624) (19.0113, -21.9176) (19.0271, -21.973) (19.0426, -22.0285) (19.0579, -22.0842) (19.0729, -22.1399) (19.0877, -22.1959) (19.1023, -22.2519) (19.1166, -22.3081) (19.1307, -22.3645) (19.1446, -22.4209) (19.1582, -22.4775) (19.1716, -22.5342) (19.1848, -22.591) (19.1977, -22.648) (19.2104, -22.7051) (19.2229, -22.7623) (19.2352, -22.8196) (19.2473, -22.877) (19.2567, -22.923) (19.2637, -22.9576) (19.2683, -22.9807) (19.2706, -22.9922) knots 0 0 0 0 0 0 0.01428571 0.02857143 0.04285714 0.05714286 0.07142857 0.08571429 0.1 0.11428571 0.12857143 0.14285714 0.15714286 0.17142857 0.18571429 0.2 0.21428571 0.22857143 0.24285714 0.25714286 0.27142857 0.28571429 0.3 0.31428571 0.32857143 0.34285714 0.35714286 0.37142857 0.38571429 0.4 0.41428571 0.42857143 0.44285714 0.45714286 0.47142857 0.48571429 0.5 0.51428571 0.52857143 0.54285714 0.55714286 0.57142857 0.58571429 0.6 0.61428571 0.62857143 0.64285714 0.65714286 0.67142857 0.68571429 0.7 0.71428571 0.72857143 0.74285714 0.75714286 0.77142857 0.78571429 0.8 0.81428571 0.82857143 0.84285714 0.85714286 0.87142857 0.88571429 0.9 0.91428571 0.92857143 0.94285714 0.95714286 0.97142857 0.98571429 1 1 1 1 1 1
  line L45 (17.823, -19.3554) -> (17.3993, -18.8953)
  arc A47 (17.3993, -18.8953) -> (18.8953, -17.3993) centre (0, 0) ccw
  line L46 (18.8953, -17.3993) -> (19.3554, -17.823)
  spline S46 degree 5 poles (19.3554, -17.823) (19.3633, -17.8303) (19.3794, -17.8447) (19.404, -17.8658) (19.4377, -17.8927) (19.4812, -17.9248) (19.5255, -17.9558) (19.5705, -17.9861) (19.6158, -18.016) (19.6613, -18.0457) (19.7071, -18.0752) (19.7531, -18.1042) (19.7995, -18.1329) (19.8463, -18.1609) (19.8936, -18.1884) (19.9412, -18.2154) (19.9893, -18.242) (20.0376, -18.2682) (20.0861, -18.294) (20.1349, -18.3196) (20.1839, -18.3448) (20.2332, -18.3698) (20.2827, -18.3943) (20.3324, -18.4186) (20.3825, -18.4425) (20.4327, -18.466) (20.4832, -18.4892) (20.534, -18.5121) (20.5849, -18.5348) (20.636, -18.5571) (20.6874, -18.5792) (20.7389, -18.6009) (20.7906, -18.6224) (20.8426, -18.6436) (20.8947, -18.6645) (20.947, -18.6851) (20.9995, -18.7054) (21.0522, -18.7255) (21.105, -18.7453) (21.1581, -18.7648) (21.2113, -18.7841) (21.2647, -18.8031) (21.3182, -18.8218) (21.3719, -18.8403) (21.4258, -18.8585) (21.4798, -18.8765) (21.534, -18.8942) (21.5884, -18.9117) (21.6429, -18.9289) (21.6975, -18.9459) (21.7523, -18.9626) (21.8073, -18.9791) (21.8624, -18.9953) (21.9176, -19.0113) (21.973, -19.0271) (22.0285, -19.0426) (22.0842, -19.0579) (22.1399, -19.0729) (22.1959, -19.0877) (22.2519, -19.1023) (22.3081, -19.1166) (22.3645, -19.1307) (22.4209, -19.1446) (22.4775, -19.1582) (22.5342, -19.1716) (22.591, -19.1848) (22.648, -19.1977) (22.7051, -19.2104) (22.7623, -19.2229) (22.8196, -19.2352) (22.877, -19.2473) (22.923, -19.2567) (22.9576, -19.2637) (22.9807, -19.2683) (22.9922, -19.2706) knots 0 0 0 0 0 0 0.01428571 0.02857143 0.04285714 0.05714286 0.07142857 0.08571429 0.1 0.11428571 0.12857143 0.14285714 0.15714286 0.17142857 0.18571429 0.2 0.21428571 0.22857143 0.24285714 0.25714286 0.27142857 0.28571429 0.3 0.31428571 0.32857143 0.34285714 0.35714286 0.37142857 0.38571429 0.4 0.41428571 0.42857143 0.44285714 0.45714286 0.47142857 0.48571429 0.5 0.51428571 0.52857143 0.54285714 0.55714286 0.57142857 0.58571429 0.6 0.61428571 0.62857143 0.64285714 0.65714286 0.67142857 0.68571429 0.7 0.71428571 0.72857143 0.74285714 0.75714286 0.77142857 0.78571429 0.8 0.81428571 0.82857143 0.84285714 0.85714286 0.87142857 0.88571429 0.9 0.91428571 0.92857143 0.94285714 0.95714286 0.97142857 0.98571429 1 1 1 1 1 1
  arc A48 (22.9922, -19.2706) -> (23.9037, -18.1277) centre (0, 0) ccw
  spline S47 degree 5 poles (21.6831, -14.9041) (21.692, -14.9103) (21.7096, -14.9227) (21.7356, -14.942) (21.7694, -14.9689) (21.8104, -15.0041) (21.8505, -15.0405) (21.89, -15.0776) (21.9293, -15.1151) (21.9683, -15.1528) (22.0072, -15.1909) (22.0458, -15.2293) (22.084, -15.2681) (22.1218, -15.3075) (22.1592, -15.3475) (22.1961, -15.388) (22.2327, -15.4289) (22.2689, -15.4701) (22.3049, -15.5117) (22.3407, -15.5536) (22.3762, -15.5958) (22.4115, -15.6382) (22.4465, -15.681) (22.4812, -15.7242) (22.5156, -15.7676) (22.5497, -15.8114) (22.5836, -15.8554) (22.6172, -15.8998) (22.6506, -15.9444) (22.6838, -15.9893) (22.7167, -16.0344) (22.7494, -16.0798) (22.7818, -16.1255) (22.814, -16.1714) (22.846, -16.2176) (22.8777, -16.264) (22.9093, -16.3107) (22.9405, -16.3576) (22.9716, -16.4047) (23.0025, -16.452) (23.0331, -16.4996) (23.0635, -16.5474) (23.0937, -16.5955) (23.1237, -16.6437) (23.1534, -16.6922) (23.183, -16.7409) (23.2123, -16.7897) (23.2414, -16.8388) (23.2703, -16.8881) (23.299, -16.9377) (23.3275, -16.9874) (23.3558, -17.0373) (23.3839, -17.0874) (23.4118, -17.1377) (23.4395, -17.1881) (23.467, -17.2388) (23.4942, -17.2897) (23.5213, -17.3407) (23.5482, -17.392) (23.5749, -17.4434) (23.6013, -17.495) (23.6276, -17.5468) (23.6537, -17.5987) (23.6796, -17.6508) (23.7053, -17.7031) (23.7308, -17.7556) (23.7561, -17.8083) (23.7812, -17.8611) (23.8061, -17.9141) (23.8308, -17.9672) (23.8553, -18.0205) (23.8748, -18.0633) (23.8893, -18.0954) (23.8989, -18.1169) (23.9037, -18.1277) knots 0 0 0 0 0 0 0.01428571 0.02857143 0.04285714 0.05714286 0.07142857 0.08571429 0.1 0.11428571 0.12857143 0.14285714 0.15714286 0.17142857 0.18571429 0.2 0.21428571 0.22857143 0.24285714 0.25714286 0.27142857 0.28571429 0.3 0.31428571 0.32857143 0.34285714 0.35714286 0.37142857 0.38571429 0.4 0.41428571 0.42857143 0.44285714 0.45714286 0.47142857 0.48571429 0.5 0.51428571 0.52857143 0.54285714 0.55714286 0.57142857 0.58571429 0.6 0.61428571 0.62857143 0.64285714 0.65714286 0.67142857 0.68571429 0.7 0.71428571 0.72857143 0.74285714 0.75714286 0.77142857 0.78571429 0.8 0.81428571 0.82857143 0.84285714 0.85714286 0.87142857 0.88571429 0.9 0.91428571 0.92857143 0.94285714 0.95714286 0.97142857 0.98571429 1 1 1 1 1 1
  line L47 (21.6831, -14.9041) -> (21.1677, -14.5499)
  arc A49 (21.1677, -14.5499) -> (22.2933, -12.7585) centre (0, 0) ccw
  line L48 (22.2933, -12.7585) -> (22.8361, -13.0691)
  spline S48 degree 5 poles (22.8361, -13.0691) (22.8455, -13.0745) (22.8643, -13.085) (22.893, -13.1) (22.9319, -13.1188) (22.9814, -13.1404) (23.0315, -13.1608) (23.0821, -13.1803) (23.133, -13.1994) (23.1839, -13.2182) (23.2351, -13.2367) (23.2864, -13.2548) (23.338, -13.2724) (23.3899, -13.2894) (23.4421, -13.3057) (23.4946, -13.3214) (23.5473, -13.3366) (23.6002, -13.3514) (23.6533, -13.3658) (23.7066, -13.3798) (23.76, -13.3935) (23.8135, -13.4069) (23.8673, -13.4198) (23.9212, -13.4324) (23.9753, -13.4445) (24.0295, -13.4563) (24.0839, -13.4677) (24.1385, -13.4788) (24.1932, -13.4895) (24.248, -13.4999) (24.3029, -13.51) (24.358, -13.5197) (24.4132, -13.5291) (24.4686, -13.5382) (24.524, -13.547) (24.5796, -13.5555) (24.6353, -13.5636) (24.6912, -13.5714) (24.7471, -13.579) (24.8032, -13.5862) (24.8593, -13.5932) (24.9156, -13.5998) (24.972, -13.6062) (25.0284, -13.6123) (25.085, -13.618) (25.1417, -13.6235) (25.1985, -13.6288) (25.2553, -13.6337) (25.3123, -13.6383) (25.3694, -13.6427) (25.4265, -13.6468) (25.4838, -13.6507) (25.5411, -13.6542) (25.5985, -13.6575) (25.656, -13.6606) (25.7136, -13.6633) (25.7712, -13.6659) (25.829, -13.6681) (25.8868, -13.6701) (25.9447, -13.6718) (26.0027, -13.6733) (26.0607, -13.6745) (26.1188, -13.6754) (26.177, -13.6761) (26.2353, -13.6766) (26.2936, -13.6768) (26.3521, -13.6767) (26.4105, -13.6765) (26.4691, -13.6759) (26.5277, -13.6751) (26.5863, -13.6741) (26.6333, -13.6731) (26.6686, -13.6722) (26.6921, -13.6715) (26.7039, -13.6712) knots 0 0 0 0 0 0 0.01428571 0.02857143 0.04285714 0.05714286 0.07142857 0.08571429 0.1 0.11428571 0.12857143 0.14285714 0.15714286 0.17142857 0.18571429 0.2 0.21428571 0.22857143 0.24285714 0.25714286 0.27142857 0.28571429 0.3 0.31428571 0.32857143 0.34285714 0.35714286 0.37142857 0.38571429 0.4 0.41428571 0.42857143 0.44285714 0.45714286 0.47142857 0.48571429 0.5 0.51428571 0.52857143 0.54285714 0.55714286 0.57142857 0.58571429 0.6 0.61428571 0.62857143 0.64285714 0.65714286 0.67142857 0.68571429 0.7 0.71428571 0.72857143 0.74285714 0.75714286 0.77142857 0.78571429 0.8 0.81428571 0.82857143 0.84285714 0.85714286 0.87142857 0.88571429 0.9 0.91428571 0.92857143 0.94285714 0.95714286 0.97142857 0.98571429 1 1 1 1 1 1
  arc A50 (26.7039, -13.6712) -> (27.3382, -12.3541) centre (0, 0) ccw
  spline S49 degree 5 poles (24.4559, -9.7055) (24.466, -9.7095) (24.4859, -9.7177) (24.5156, -9.7307) (24.5545, -9.7494) (24.6023, -9.7746) (24.6494, -9.8012) (24.6963, -9.8286) (24.7429, -9.8564) (24.7894, -9.8845) (24.8357, -9.9129) (24.8819, -9.9418) (24.9278, -9.9712) (24.9734, -10.0012) (25.0187, -10.0318) (25.0637, -10.0631) (25.1085, -10.0948) (25.153, -10.127) (25.1974, -10.1595) (25.2416, -10.1924) (25.2856, -10.2256) (25.3294, -10.2591) (25.3731, -10.2931) (25.4165, -10.3274) (25.4597, -10.3621) (25.5027, -10.3972) (25.5456, -10.4326) (25.5882, -10.4683) (25.6307, -10.5044) (25.673, -10.5408) (25.7151, -10.5775) (25.7571, -10.6145) (25.7989, -10.6518) (25.8405, -10.6894) (25.882, -10.7273) (25.9232, -10.7654) (25.9643, -10.8039) (26.0053, -10.8427) (26.0461, -10.8817) (26.0867, -10.921) (26.1271, -10.9606) (26.1674, -11.0004) (26.2075, -11.0406) (26.2475, -11.0809) (26.2873, -11.1216) (26.3269, -11.1624) (26.3664, -11.2036) (26.4057, -11.245) (26.4449, -11.2866) (26.4839, -11.3285) (26.5227, -11.3706) (26.5614, -11.4129) (26.5999, -11.4555) (26.6383, -11.4984) (26.6765, -11.5414) (26.7146, -11.5847) (26.7525, -11.6282) (26.7902, -11.672) (26.8279, -11.716) (26.8653, -11.7601) (26.9026, -11.8046) (26.9397, -11.8492) (26.9767, -11.894) (27.0136, -11.9391) (27.0502, -11.9844) (27.0868, -12.0299) (27.1231, -12.0755) (27.1594, -12.1215) (27.1954, -12.1676) (27.2314, -12.2139) (27.2671, -12.2604) (27.2956, -12.2978) (27.3169, -12.3259) (27.3311, -12.3447) (27.3382, -12.3541) knots 0 0 0 0 0 0 0.01428571 0.02857143 0.04285714 0.05714286 0.07142857 0.08571429 0.1 0.11428571 0.12857143 0.14285714 0.15714286 0.17142857 0.18571429 0.2 0.21428571 0.22857143 0.24285714 0.25714286 0.27142857 0.28571429 0.3 0.31428571 0.32857143 0.34285714 0.35714286 0.37142857 0.38571429 0.4 0.41428571 0.42857143 0.44285714 0.45714286 0.47142857 0.48571429 0.5 0.51428571 0.52857143 0.54285714 0.55714286 0.57142857 0.58571429 0.6 0.61428571 0.62857143 0.64285714 0.65714286 0.67142857 0.68571429 0.7 0.71428571 0.72857143 0.74285714 0.75714286 0.77142857 0.78571429 0.8 0.81428571 0.82857143 0.84285714 0.85714286 0.87142857 0.88571429 0.9 0.91428571 0.92857143 0.94285714 0.95714286 0.97142857 0.98571429 1 1 1 1 1 1
  line L49 (24.4559, -9.7055) -> (23.8746, -9.4748)
  arc A51 (23.8746, -9.4748) -> (24.5734, -7.4779) centre (0, 0) ccw
  line L50 (24.5734, -7.4779) -> (25.1717, -7.6599)
  spline S50 degree 5 poles (25.1717, -7.6599) (25.182, -7.6631) (25.2028, -7.6691) (25.2341, -7.6774) (25.2761, -7.6871) (25.3292, -7.6971) (25.3826, -7.7058) (25.4363, -7.7136) (25.4901, -7.7209) (25.544, -7.7279) (25.598, -7.7346) (25.6521, -7.7408) (25.7063, -7.7465) (25.7606, -7.7514) (25.8152, -7.7557) (25.8698, -7.7594) (25.9246, -7.7625) (25.9795, -7.7651) (26.0345, -7.7673) (26.0895, -7.7692) (26.1446, -7.7706) (26.1998, -7.7717) (26.2551, -7.7724) (26.3104, -7.7726) (26.3659, -7.7725) (26.4214, -7.7719) (26.4769, -7.7709) (26.5326, -7.7695) (26.5883, -7.7678) (26.644, -7.7657) (26.6999, -7.7633) (26.7557, -7.7606) (26.8117, -7.7575) (26.8676, -7.754) (26.9237, -7.7502) (26.9797, -7.7461) (27.0359, -7.7417) (27.092, -7.7369) (27.1483, -7.7318) (27.2045, -7.7264) (27.2608, -7.7206) (27.3172, -7.7146) (27.3735, -7.7083) (27.4299, -7.7016) (27.4864, -7.6947) (27.5429, -7.6874) (27.5994, -7.6799) (27.6559, -7.672) (27.7125, -7.6639) (27.7691, -7.6555) (27.8257, -7.6468) (27.8824, -7.6378) (27.9391, -7.6285) (27.9958, -7.6189) (28.0525, -7.6091) (28.1093, -7.599) (28.166, -7.5886) (28.2228, -7.5779) (28.2796, -7.567) (28.3365, -7.5558) (28.3933, -7.5443) (28.4502, -7.5326) (28.5071, -7.5206) (28.564, -7.5083) (28.6209, -7.4958) (28.6778, -7.483) (28.7347, -7.47) (28.7917, -7.4567) (28.8486, -7.4431) (28.9056, -7.4293) (28.9625, -7.4152) (29.0081, -7.4038) (29.0423, -7.3951) (29.0651, -7.3892) (29.0765, -7.3863) knots 0 0 0 0 0 0 0.01428571 0.02857143 0.04285714 0.05714286 0.07142857 0.08571429 0.1 0.11428571 0.12857143 0.14285714 0.15714286 0.17142857 0.18571429 0.2 0.21428571 0.22857143 0.24285714 0.25714286 0.27142857 0.28571429 0.3 0.31428571 0.32857143 0.34285714 0.35714286 0.37142857 0.38571429 0.4 0.41428571 0.42857143 0.44285714 0.45714286 0.47142857 0.48571429 0.5 0.51428571 0.52857143 0.54285714 0.55714286 0.57142857 0.58571429 0.6 0.61428571 0.62857143 0.64285714 0.65714286 0.67142857 0.68571429 0.7 0.71428571 0.72857143 0.74285714 0.75714286 0.77142857 0.78571429 0.8 0.81428571 0.82857143 0.84285714 0.85714286 0.87142857 0.88571429 0.9 0.91428571 0.92857143 0.94285714 0.95714286 0.97142857 0.98571429 1 1 1 1 1 1
  arc A52 (29.0765, -7.3863) -> (29.4018, -5.961) centre (0, 0) ccw
  spline S51 degree 5 poles (26.0024, -4.0202) (26.0131, -4.0219) (26.0344, -4.0254) (26.0662, -4.0315) (26.1083, -4.0411) (26.1605, -4.055) (26.2124, -4.0704) (26.2641, -4.0867) (26.3158, -4.1034) (26.3674, -4.1205) (26.4189, -4.1379) (26.4703, -4.1558) (26.5216, -4.1742) (26.5728, -4.1933) (26.6237, -4.2131) (26.6746, -4.2336) (26.7253, -4.2545) (26.7759, -4.276) (26.8263, -4.2978) (26.8767, -4.32) (26.927, -4.3426) (26.9772, -4.3656) (27.0273, -4.389) (27.0773, -4.4128) (27.1272, -4.437) (27.1769, -4.4616) (27.2266, -4.4866) (27.2761, -4.512) (27.3255, -4.5377) (27.3749, -4.5637) (27.4241, -4.5901) (27.4733, -4.6168) (27.5223, -4.6439) (27.5712, -4.6713) (27.6201, -4.699) (27.6688, -4.7271) (27.7175, -4.7554) (27.766, -4.7841) (27.8144, -4.8131) (27.8628, -4.8424) (27.911, -4.872) (27.9591, -4.9018) (28.0072, -4.932) (28.0551, -4.9625) (28.103, -4.9932) (28.1507, -5.0243) (28.1983, -5.0556) (28.2459, -5.0872) (28.2933, -5.1191) (28.3407, -5.1512) (28.3879, -5.1836) (28.4351, -5.2163) (28.4821, -5.2493) (28.529, -5.2825) (28.5759, -5.316) (28.6226, -5.3497) (28.6693, -5.3837) (28.7158, -5.418) (28.7623, -5.4525) (28.8086, -5.4872) (28.8548, -5.5222) (28.901, -5.5574) (28.947, -5.5929) (28.993, -5.6287) (29.0388, -5.6647) (29.0845, -5.7009) (29.1302, -5.7373) (29.1757, -5.774) (29.2211, -5.8109) (29.2665, -5.8481) (29.3117, -5.8855) (29.3478, -5.9156) (29.3748, -5.9383) (29.3928, -5.9534) (29.4018, -5.961) knots 0 0 0 0 0 0 0.01428571 0.02857143 0.04285714 0.05714286 0.07142857 0.08571429 0.1 0.11428571 0.12857143 0.14285714 0.15714286 0.17142857 0.18571429 0.2 0.21428571 0.22857143 0.24285714 0.25714286 0.27142857 0.28571429 0.3 0.31428571 0.32857143 0.34285714 0.35714286 0.37142857 0.38571429 0.4 0.41428571 0.42857143 0.44285714 0.45714286 0.47142857 0.48571429 0.5 0.51428571 0.52857143 0.54285714 0.55714286 0.57142857 0.58571429 0.6 0.61428571 0.62857143 0.64285714 0.65714286 0.67142857 0.68571429 0.7 0.71428571 0.72857143 0.74285714 0.75714286 0.77142857 0.78571429 0.8 0.81428571 0.82857143 0.84285714 0.85714286 0.87142857 0.88571429 0.9 0.91428571 0.92857143 0.94285714 0.95714286 0.97142857 0.98571429 1 1 1 1 1 1
  line L51 (26.0024, -4.0202) -> (25.3844, -3.9247)
  arc A53 (25.3844, -3.9247) -> (25.6213, -1.8223) centre (0, 0) ccw
  line L52 (25.6213, -1.8223) -> (26.2451, -1.8667)
  spline S52 degree 5 poles (26.2451, -1.8667) (26.2559, -1.8674) (26.2774, -1.8687) (26.3098, -1.8698) (26.3529, -1.8699) (26.4069, -1.8679) (26.461, -1.8644) (26.515, -1.8601) (26.5691, -1.8552) (26.6232, -1.8501) (26.6773, -1.8446) (26.7314, -1.8386) (26.7855, -1.8321) (26.8396, -1.8248) (26.8937, -1.8169) (26.9478, -1.8082) (27.0019, -1.7991) (27.056, -1.7894) (27.1101, -1.7794) (27.1642, -1.7689) (27.2182, -1.7581) (27.2723, -1.7469) (27.3263, -1.7352) (27.3803, -1.7231) (27.4343, -1.7106) (27.4883, -1.6977) (27.5423, -1.6844) (27.5962, -1.6707) (27.6502, -1.6566) (27.7041, -1.6422) (27.7579, -1.6274) (27.8118, -1.6123) (27.8656, -1.5968) (27.9194, -1.581) (27.9732, -1.5648) (28.027, -1.5483) (28.0807, -1.5315) (28.1344, -1.5143) (28.1881, -1.4969) (28.2417, -1.4791) (28.2953, -1.461) (28.3489, -1.4425) (28.4025, -1.4238) (28.456, -1.4048) (28.5095, -1.3854) (28.5629, -1.3658) (28.6163, -1.3459) (28.6697, -1.3256) (28.7231, -1.3051) (28.7764, -1.2843) (28.8296, -1.2632) (28.8829, -1.2418) (28.9361, -1.2202) (28.9892, -1.1983) (29.0423, -1.176) (29.0954, -1.1536) (29.1485, -1.1308) (29.2015, -1.1078) (29.2544, -1.0845) (29.3073, -1.0609) (29.3602, -1.0371) (29.413, -1.013) (29.4658, -0.9886) (29.5186, -0.964) (29.5712, -0.9391) (29.6239, -0.914) (29.6765, -0.8886) (29.729, -0.863) (29.7816, -0.8371) (29.834, -0.8109) (29.8864, -0.7845) (29.9283, -0.7632) (29.9597, -0.7471) (29.9806, -0.7364) (29.9911, -0.731) knots 0 0 0 0 0 0 0.01428571 0.02857143 0.04285714 0.05714286 0.07142857 0.08571429 0.1 0.11428571 0.12857143 0.14285714 0.15714286 0.17142857 0.18571429 0.2 0.21428571 0.22857143 0.24285714 0.25714286 0.27142857 0.28571429 0.3 0.31428571 0.32857143 0.34285714 0.35714286 0.37142857 0.38571429 0.4 0.41428571 0.42857143 0.44285714 0.45714286 0.47142857 0.48571429 0.5 0.51428571 0.52857143 0.54285714 0.55714286 0.57142857 0.58571429 0.6 0.61428571 0.62857143 0.64285714 0.65714286 0.67142857 0.68571429 0.7 0.71428571 0.72857143 0.74285714 0.75714286 0.77142857 0.78571429 0.8 0.81428571 0.82857143 0.84285714 0.85714286 0.87142857 0.88571429 0.9 0.91428571 0.92857143 0.94285714 0.95714286 0.97142857 0.98571429 1 1 1 1 1 1
  arc A54 (29.9911, -0.731) -> (29.9911, 0.731) centre (0, 0) ccw
  spline S53 degree 5 poles (26.2451, 1.8667) (26.2559, 1.8674) (26.2774, 1.8687) (26.3098, 1.8698) (26.3529, 1.8699) (26.4069, 1.8679) (26.461, 1.8644) (26.515, 1.8601) (26.5691, 1.8552) (26.6232, 1.8501) (26.6773, 1.8446) (26.7314, 1.8386) (26.7855, 1.8321) (26.8396, 1.8248) (26.8937, 1.8169) (26.9478, 1.8082) (27.0019, 1.7991) (27.056, 1.7894) (27.1101, 1.7794) (27.1642, 1.7689) (27.2182, 1.7581) (27.2723, 1.7469) (27.3263, 1.7352) (27.3803, 1.7231) (27.4343, 1.7106) (27.4883, 1.6977) (27.5423, 1.6844) (27.5962, 1.6707) (27.6502, 1.6566) (27.7041, 1.6422) (27.7579, 1.6274) (27.8118, 1.6123) (27.8656, 1.5968) (27.9194, 1.581) (27.9732, 1.5648) (28.027, 1.5483) (28.0807, 1.5315) (28.1344, 1.5143) (28.1881, 1.4969) (28.2417, 1.4791) (28.2953, 1.461) (28.3489, 1.4425) (28.4025, 1.4238) (28.456, 1.4048) (28.5095, 1.3854) (28.5629, 1.3658) (28.6163, 1.3459) (28.6697, 1.3256) (28.7231, 1.3051) (28.7764, 1.2843) (28.8296, 1.2632) (28.8829, 1.2418) (28.9361, 1.2202) (28.9892, 1.1983) (29.0423, 1.176) (29.0954, 1.1536) (29.1485, 1.1308) (29.2015, 1.1078) (29.2544, 1.0845) (29.3073, 1.0609) (29.3602, 1.0371) (29.413, 1.013) (29.4658, 0.9886) (29.5186, 0.964) (29.5712, 0.9391) (29.6239, 0.914) (29.6765, 0.8886) (29.729, 0.863) (29.7816, 0.8371) (29.834, 0.8109) (29.8864, 0.7845) (29.9283, 0.7632) (29.9597, 0.7471) (29.9806, 0.7364) (29.9911, 0.731) knots 0 0 0 0 0 0 0.01428571 0.02857143 0.04285714 0.05714286 0.07142857 0.08571429 0.1 0.11428571 0.12857143 0.14285714 0.15714286 0.17142857 0.18571429 0.2 0.21428571 0.22857143 0.24285714 0.25714286 0.27142857 0.28571429 0.3 0.31428571 0.32857143 0.34285714 0.35714286 0.37142857 0.38571429 0.4 0.41428571 0.42857143 0.44285714 0.45714286 0.47142857 0.48571429 0.5 0.51428571 0.52857143 0.54285714 0.55714286 0.57142857 0.58571429 0.6 0.61428571 0.62857143 0.64285714 0.65714286 0.67142857 0.68571429 0.7 0.71428571 0.72857143 0.74285714 0.75714286 0.77142857 0.78571429 0.8 0.81428571 0.82857143 0.84285714 0.85714286 0.87142857 0.88571429 0.9 0.91428571 0.92857143 0.94285714 0.95714286 0.97142857 0.98571429 1 1 1 1 1 1
  line L53 (26.2451, 1.8667) -> (25.6213, 1.8223)
  arc A55 (25.6213, 1.8223) -> (25.3844, 3.9247) centre (0, 0) ccw
  line L54 (25.3844, 3.9247) -> (26.0024, 4.0202)
  spline S54 degree 5 poles (26.0024, 4.0202) (26.0131, 4.0219) (26.0344, 4.0254) (26.0662, 4.0315) (26.1083, 4.0411) (26.1605, 4.055) (26.2124, 4.0704) (26.2641, 4.0867) (26.3158, 4.1034) (26.3674, 4.1205) (26.4189, 4.1379) (26.4703, 4.1558) (26.5216, 4.1742) (26.5728, 4.1933) (26.6237, 4.2131) (26.6746, 4.2336) (26.7253, 4.2545) (26.7759, 4.276) (26.8263, 4.2978) (26.8767, 4.32) (26.927, 4.3426) (26.9772, 4.3656) (27.0273, 4.389) (27.0773, 4.4128) (27.1272, 4.437) (27.1769, 4.4616) (27.2266, 4.4866) (27.2761, 4.512) (27.3255, 4.5377) (27.3749, 4.5637) (27.4241, 4.5901) (27.4733, 4.6168) (27.5223, 4.6439) (27.5712, 4.6713) (27.6201, 4.699) (27.6688, 4.7271) (27.7175, 4.7554) (27.766, 4.7841) (27.8144, 4.8131) (27.8628, 4.8424) (27.911, 4.872) (27.9591, 4.9018) (28.0072, 4.932) (28.0551, 4.9625) (28.103, 4.9932) (28.1507, 5.0243) (28.1983, 5.0556) (28.2459, 5.0872) (28.2933, 5.1191) (28.3407, 5.1512) (28.3879, 5.1836) (28.4351, 5.2163) (28.4821, 5.2493) (28.529, 5.2825) (28.5759, 5.316) (28.6226, 5.3497) (28.6693, 5.3837) (28.7158, 5.418) (28.7623, 5.4525) (28.8086, 5.4872) (28.8548, 5.5222) (28.901, 5.5574) (28.947, 5.5929) (28.993, 5.6287) (29.0388, 5.6647) (29.0845, 5.7009) (29.1302, 5.7373) (29.1757, 5.774) (29.2211, 5.8109) (29.2665, 5.8481) (29.3117, 5.8855) (29.3478, 5.9156) (29.3748, 5.9383) (29.3928, 5.9534) (29.4018, 5.961) knots 0 0 0 0 0 0 0.01428571 0.02857143 0.04285714 0.05714286 0.07142857 0.08571429 0.1 0.11428571 0.12857143 0.14285714 0.15714286 0.17142857 0.18571429 0.2 0.21428571 0.22857143 0.24285714 0.25714286 0.27142857 0.28571429 0.3 0.31428571 0.32857143 0.34285714 0.35714286 0.37142857 0.38571429 0.4 0.41428571 0.42857143 0.44285714 0.45714286 0.47142857 0.48571429 0.5 0.51428571 0.52857143 0.54285714 0.55714286 0.57142857 0.58571429 0.6 0.61428571 0.62857143 0.64285714 0.65714286 0.67142857 0.68571429 0.7 0.71428571 0.72857143 0.74285714 0.75714286 0.77142857 0.78571429 0.8 0.81428571 0.82857143 0.84285714 0.85714286 0.87142857 0.88571429 0.9 0.91428571 0.92857143 0.94285714 0.95714286 0.97142857 0.98571429 1 1 1 1 1 1
  arc A56 (29.4018, 5.961) -> (29.0765, 7.3863) centre (0, 0) ccw